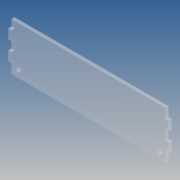
# Autodesk Inventor part: KB33-046-004-014 - Лицевая вертикальня пластина
Saved by Autodesk Inventor 2020 (Build 240168000, 168)
## iProperties
Created: 2021-06-26
Part Number: KB33-046-004-014 - Лицевая вертикальня пластина
Material: Пластик ПЭТ
Document SubType Name: Modeling
Designer: Петров Иван
Mass: 73.1479 g
Surface Area: 260.024 cm^2
Volume: 47.4678 cm^3
Density: 1.541 g/cm^3
Appearance: Поликарбонат — прозрачный
Author: Петров Иван
Autodesk Inventor part; units mm, degrees
ref_plane "YZ Plane" through (0, 0, 0) normal (1, 0, 0) x (0, 1, 0)
ref_plane "XZ Plane" through (0, 0, 0) normal (0, 1, 0) x (-1, 0, 0)
ref_plane "XY Plane" through (0, 0, 0) normal (0, 0, 1) x (1, 0, 0)
sketch "Эскиз1" plane through (0, 0, 0) normal (0, 0, 1) x (1, 0, 0)
  line L0 (-26.3955, 0) -> (-26.3955, 30) projected
  line L1 (168.6045, 0) -> (168.6045, 30) projected
  circle A0 centre (161.1045, 7.5) radius 2 projected
  circle A1 centre (-18.8955, 7.5) radius 2 projected
  line L2 (-26.3955, 60.0004) -> (-30.3955, 60.0004) projected
  line L3 (172.6045, 60.0004) -> (168.6045, 60.0004) projected
  line L4 (-26.3955, 60.0004) -> (168.6045, 60.0004)
  line L5 (168.6045, 60.0004) -> (168.6045, 0)
  line L6 (168.6045, 0) -> (-26.3955, 0)
  line L7 (-26.3955, 0) -> (-26.3955, 60.0004)
  point P0 (0, 0)
  constraints: 8 end point, 2 parallel, 1 horizontal, 1 perpendicular
extrude "Выдавливание1" add sketch "Эскиз1" along normal blind 4
thicken "Толщина1" operation add thickness 4 both sides no extend neighbours yes toward (1, 0, 0) faces at (168.6045, 10, 1.3333)
thicken "Толщина2" operation add thickness 4 both sides no extend neighbours yes toward (-1, 0, 0) faces at (-26.3955, 40.0003, 2.6667)
sketch "Эскиз2" plane through (0, 0, 4) normal (0, 0, 1) x (1, 0, 0)
  line L0 (172.6045, 60.0004) -> (-30.3955, 60.0004) projected
  line L1 (-30.3955, 60.0004) -> (-26.3955, 60.0004)
  line L2 (-26.3955, 60.0004) -> (-26.3955, 48.0004)
  line L3 (-26.3955, 48.0004) -> (-30.3955, 48.0004)
  line L4 (-30.3955, 48.0004) -> (-30.3955, 60.0004)
  line L5 (172.6045, 60.0004) -> (168.6045, 60.0004)
  line L6 (168.6045, 60.0004) -> (168.6045, 48.0004)
  line L7 (168.6045, 48.0004) -> (172.6045, 48.0004)
  line L8 (172.6045, 48.0004) -> (172.6045, 60.0004)
  point P0 (0, 0)
  dimension "d6" = 4
  dimension "d7" = 12
  dimension "d8" = 4
  dimension "d9" = 12
  constraints: 16 end point, 4 parallel, 2 horizontal, 2 perpendicular
  measures "d6" distance of L2.end L3.end
  measures "d7" distance of L1.end L2.end
  measures "d8" distance of L7.end L6.end
  measures "d9" distance of L6.end L5.end
extrude "Выдавливание2" cut sketch "Эскиз2" against normal blind 4
pattern_linear "Прямоуг.массив1" count 3 spacing 24 along (0, -1, 0) of "Выдавливание2"
thicken "Толщина3" operation add thickness 4 both sides no extend neighbours yes toward (1, 0, 0) faces at (-30.3955, 0.0003, 1.3333) (-29.0622, 0.0004, 2.6667)
thicken "Толщина4" operation add thickness 4 both sides no extend neighbours yes toward (-1, 0, 0) faces at (172.6045, 0.0001, 1.3333) (169.9378, 0.0004, 2.6667)
